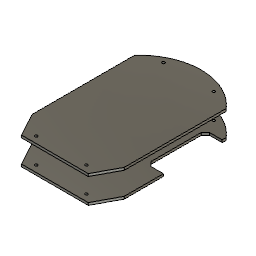
chassis (Autodesk Fusion 360 design; units mm, degrees)
Autodesk Fusion 360 part; units mm, degrees
sketch "Sketch1" plane through (0, 0, 0) normal (0, 0, 1) x (1, 0, 0)
  line L0 (55, 149.9202) -> (55, 28)
  line L1 (40, 0) -> (-40, 0)
  line L2 (-55, 28) -> (-55, 149.9202)
  arc A0 (55, 149.9202) -> (-55, 149.9202) centre (0, 102.1526) ccw
  line L3 (55, 28) -> (40, 0)
  line L4 (-40, 0) -> (-55, 28)
  line L5 (0, 175) -> (1.8351, 175) construction
  line L6 (1.8351, 175) -> (80, 175) construction
  point P0 (55, 0)
  point P1 (-55, 0)
  dimension "d3" = 72.8474
  dimension "d4" = 28
  dimension "d5" = 15
  dimension "d6" = 15
  dimension "d7" = 28
  dimension "d8" = 175
  dimension "d9" = 121.9202
  constraint vertical L0
  constraint horizontal L1
  constraint vertical L2
  constraint horizontal L2.end L0.start
  constraint coincident origin L1
  constraint coincident P0 L0
  constraint coincident P0 L1
  constraint coincident P1 L1
  constraint coincident P1 L2
  constraint midpoint A0 L5.start
  constraint tangent A0 L5
  constraint horizontal L5
  constraint parallel L5 L6
  measures "d3" radius of A0
  measures "d4" distance of P0 L0.end
  measures "d5" distance of P0 L1.start
  measures "d6" distance of P1 L1.end
  measures "d7" distance of P1 L2.start
  measures "d8" distance of L1 L6
  measures "d9" distance of L0.start L0.end
sketch "Sketch2" plane through (0, 0, 0) normal (0, 0, 1) x (1, 0, 0)
  line L0 (40, 0) -> (-40, 0)
  line L1 (0, 175) -> (1.8351, 175) construction
  arc A0 (55, 149.9202) -> (-55, 149.9202) centre (0, 102.1526) ccw
  line L2 (-40, 0) -> (-55, 28)
  line L3 (1.8351, 175) -> (80, 175) construction
  line L4 (55, 28) -> (40, 0)
  line L5 (-55, 145) -> (-40, 145)
  line L6 (-35, 140) -> (-35, 80)
  line L7 (-40, 75) -> (-55, 75)
  line L8 (0, 0) -> (0, 175) construction
  line L9 (-40, 145) -> (-35, 140)
  line L10 (-35, 80) -> (-40, 75)
  line L11 (35, 80) -> (40, 75)
  line L12 (40, 75) -> (55, 75)
  line L13 (55, 145) -> (40, 145)
  line L14 (35, 140) -> (35, 80)
  line L15 (40, 145) -> (35, 140)
  line L16 (-55, 28) -> (-55, 75)
  line L17 (-55, 145) -> (-55, 149.9202)
  line L18 (55, 149.9202) -> (55, 145)
  line L19 (55, 75) -> (55, 28)
  point P0 (55, 0)
  point P1 (-55, 0)
  point P2 (-35, 145)
  point P3 (-35, 75)
  point P4 (35, 145)
  point P5 (35, 75)
  dimension "d10" = 72.8474
  dimension "d11" = 28
  dimension "d12" = 15
  dimension "d13" = 15
  dimension "d14" = 28
  dimension "d15" = 175
  dimension "d16" = 121.9202
  dimension "d17" = 20
  dimension "d18" = 70
  dimension "d19" = 5
  dimension "d20" = 5
  dimension "d21" = 5
  dimension "d22" = 5
  constraint vertical L18
  constraint horizontal L0
  constraint vertical L16
  constraint horizontal A0.end A0.start
  constraint coincident L8.start L0
  constraint coincident P0 L18
  constraint coincident P0 L0
  constraint coincident P1 L0
  constraint coincident P1 L16
  constraint midpoint L1.start A0
  constraint tangent L1 A0
  constraint horizontal L1
  constraint parallel L1 L3
  constraint horizontal L5
  constraint vertical L6
  constraint horizontal L7
  constraint coincident L5.start L16
  constraint parallel L8 L18
  constraint coincident P2 L5
  constraint coincident P2 L6
  constraint coincident P3 L6
  constraint coincident P3 L7
  constraint symmetric L5.start L8 L13.start
  constraint symmetric P2 L8 P4
  constraint symmetric P3 L8 P5
  constraint symmetric L7.end L8 L12.end
  constraint symmetric L8 L5.end L13.end
  constraint symmetric L8 L6.start L14.start
  constraint symmetric L8 L6.end L11.start
  constraint symmetric L8 L7.start L11.end
  constraint collinear L16 L17
  constraint collinear L18 L19
  measures "d10" radius of A0
  measures "d11" distance of L4.start P0
  measures "d12" distance of L0.start P0
  measures "d13" distance of L0.end P1
  measures "d14" distance of L2.end P1
  measures "d15" distance of L0 L3
  measures "d16" distance of L4.start A0.start
  measures "d17" distance of L5.start P2
  measures "d18" distance of L5.start L7.end
  measures "d19" distance of P2 L5.end
  measures "d20" distance of P2 L6.start
  measures "d21" distance of P3 L6.end
  measures "d22" distance of P3 L7.start
extrude "Extrude1" add sketch "Sketch1" along normal blind 3 makes body 1
extrude "Extrude2" add sketch "Sketch2" along normal blind 3 separate body makes body 2
move_body "Move1" bodies 1 to x (1, 0, 0) y (0, 1, 0) z (0, 0, 1) at (0, 0, 30)
sketch "Sketch3" plane through (0, 0, 0) normal (0, 0, 1) x (1, 0, 0)
  circle A0 centre (-30, 7.8025) radius 1.6
  line L0 (0, 0) -> (0, 175)
  circle A1 centre (30, 7.8025) radius 1.6
  line L1 (0, 87.5) -> (46.6549, 87.5) construction
  circle A2 centre (-30, 160) radius 1.6
  circle A3 centre (30, 160) radius 1.6
  dimension "d27" = 3.2
  dimension "d28" = 60
  dimension "d30" = 60
  dimension "d31" = 30
  constraint symmetric A0 L0 A1
  constraint midpoint L0 L1.start
  constraint perpendicular L0 L1
  measures "d27" diameter of A0
  measures "d28" distance of A0.centre A1.centre
  measures "d30" distance of A2.centre A3.centre
  measures "d31" distance of L0 A3.centre
extrude "Extrude3" cut sketch "Sketch3" along normal blind 50 bodies 1 2
equation "d20 = d19"
equation "d22 = d21"
